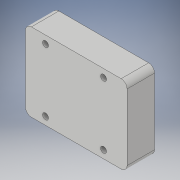
# Autodesk Inventor part: LockBooster
Saved by Autodesk Inventor 2019 (Build 230136000, 136)
## iProperties
Created: 2019-07-03
Part Number: LockBooster
Material: Generic
Document SubType Name: Modeling
Designer: garretthagen21
Density: 1 g/cm^3
Appearance: Default
Author: garretthagen21
Autodesk Inventor part; units mm, degrees
ref_plane "YZ Plane" through (0, 0, 0) normal (1, 0, 0) x (0, 1, 0)
ref_plane "XZ Plane" through (0, 0, 0) normal (0, 1, 0) x (-1, 0, 0)
ref_plane "XY Plane" through (0, 0, 0) normal (0, 0, 1) x (1, 0, 0)
sketch "Sketch1" plane through (0, 0, 0) normal (0, 0, 1) x (1, 0, 0)
  line L0 (-48.1104, 41.8216) -> (6.3726, 41.8216)
  line L1 (6.3726, 41.8216) -> (6.3726, -0.1138)
  line L2 (6.3726, -0.1138) -> (-48.1104, -0.1138)
  line L3 (-48.1104, -0.1138) -> (-48.1104, 41.8216)
  point P0 (0, 0)
  dimension "d0" = 54.483
  dimension "d1" = 41.9354
  constraints: 8 end point, 2 parallel, 1 horizontal, 1 perpendicular
  measures "d0" distance of L1.end L2.end
  measures "d1" distance of L0.end L1.end
extrude "Extrusion1" add sketch "Sketch1" along normal blind 14.732
sketch "Sketch2" plane through (0, 0, 14.732) normal (0, 0, 1) x (1, 0, 0)
  line L0 (-48.1104, 41.8216) -> (-48.1104, -0.1138) projected
  line L1 (6.3726, 41.8216) -> (-48.1104, 41.8216) projected
  line L2 (6.3726, -0.1138) -> (6.3726, 41.8216) projected
  line L3 (-48.1104, -0.1138) -> (6.3726, -0.1138) projected
  point P0 (0, 0)
  point P1 (-37.3408, 37.6306)
  point P2 (-6.2258, 37.6052)
  point P3 (-6.2258, 4.0772)
  point P4 (-37.3408, 4.0772)
  dimension "d4" = 10.7696
  dimension "d5" = 4.191
  dimension "d6" = 12.5984
  dimension "d7" = 4.191
  dimension "d16" = 4.2164
  dimension "d17" = 12.5984
  dimension "d18" = 4.191
  dimension "d19" = 10.7696
  measures "d4" distance from line of point (-37.341, 37.631) L0
  measures "d5" distance from line of point (-37.341, 37.631) L1
  measures "d6" distance from line of point (-6.226, 37.605) L2
  measures "d7" distance from line of point (-6.226, 4.077) L3
  measures "d16" distance from line of L1 point (-6.226, 37.605)
  measures "d17" distance from line of L2 point (-6.226, 4.077)
  measures "d18" distance from line of L3 point (-37.341, 4.077)
  measures "d19" distance from line of L0 point (-37.341, 4.077)
hole "Hole1" at (-37.3408, 37.6306, 14.732) at (-6.2258, 37.6052, 14.732) at (-6.2258, 4.0772, 14.732) at (-37.3408, 4.0772, 14.732) direction (0, 0, -1) diameter 3.175 end through all
fillet "Fillet1" radius 3.175 4 edges at (-48.1104, 41.8216, 7.366) (6.3726, 41.8216, 7.366) (6.3726, -0.1138, 7.366) (-48.1104, -0.1138, 7.366)
body "Solid1"
